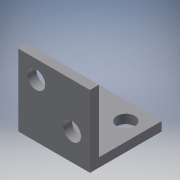
# Autodesk Inventor part: connector1by1
Saved by Autodesk Inventor 2016 (Build 200138000, 138)
## iProperties
Created: 2016-01-16
Part Number: connector1by1
Material: Generic
Document SubType Name: Modeling
Designer: Thariq
Density: 1 g/cm^3
Appearance: Default
Author: Thariq
Autodesk Inventor part; units mm, degrees
ref_plane "YZ Plane" through (0, 0, 0) normal (1, 0, 0) x (0, 1, 0)
ref_plane "XZ Plane" through (0, 0, 0) normal (0, 1, 0) x (-1, 0, 0)
ref_plane "XY Plane" through (0, 0, 0) normal (0, 0, 1) x (1, 0, 0)
sketch "Sketch1" plane through (0, 0, 0) normal (0, 1, 0) x (-1, 0, 0)
  line L0 (0, 0) -> (25.4, 0)
  line L1 (25.4, 0) -> (25.4, -25.4)
  line L2 (25.4, -25.4) -> (0, -25.4)
  line L3 (0, -25.4) -> (0, 0)
  circle A0 centre (6.35, -19.05) radius 3.175
  circle A1 centre (19.05, -9.525) radius 3.124
  line L4 (25.4, 0) -> (0, 0)
  line L5 (0, 0) -> (0, -3.175)
  line L6 (0, -3.175) -> (25.4, -3.175)
  line L7 (25.4, -3.175) -> (25.4, 0)
  dimension "d0" = 25.4
  dimension "d1" = 25.4
  dimension "d2" = 6.35
  dimension "d3" = 6.35
  dimension "d4" = 6.35
  dimension "d5" = 9.525
  dimension "d6" = 6.35
  dimension "d7" = 3.175
  constraints: 16 end point, 4 parallel, 2 centre point, 2 horizontal, 2 perpendicular, 1 point on line
  measures "d0" distance between parallel lines of L3 L1
  measures "d1" distance between parallel lines of L0 L2
  measures "d2" diameter of A0
  measures "d3" distance from line of L2 A0.centre
  measures "d4" distance from line of L3 A0.centre
  measures "d5" distance from line of L0 A1.centre
  measures "d6" distance from line of L1 A1.centre
  measures "d7" distance between parallel lines of L0 L6
extrude "Extrusion1" add sketch "Sketch1" along normal blind 3.175 contours L6 L1 L2 L3
extrude "Extrusion2" add sketch "Sketch1" along normal blind 25.4 contours L0 L1 L6 L3
sketch "Sketch2" plane through (-25.4, 0, 0) normal (0, 0, 1) x (1, 0, 0)
  circle A0 centre (6.35, 19.05) radius 3.175
  line L0 (0, 25.4) -> (25.4, 25.4) projected
  line L1 (0, 0) -> (0, 25.4) projected
  circle A1 centre (19.05, 9.525) radius 3.175
  line L2 (25.4, 0) -> (25.4, 25.4) projected
  line L3 (0, 0) -> (25.4, 0) projected
  dimension "d12" = 6.35
  dimension "d13" = 6.35
  dimension "d14" = 6.35
  dimension "d15" = 6.35
  dimension "d16" = 9.525
  dimension "d17" = 6.35
  constraints: 2 centre point
  measures "d12" distance from line of L0 A0.centre
  measures "d13" distance from line of L1 A0.centre
  measures "d14" diameter of A0
  measures "d15" distance from line of L2 A1.centre
  measures "d16" distance from line of L3 A1.centre
  measures "d17" diameter of A1
extrude "Extrusion3" cut sketch "Sketch2" against normal through all contours A0 | A1
body "Solid1"
